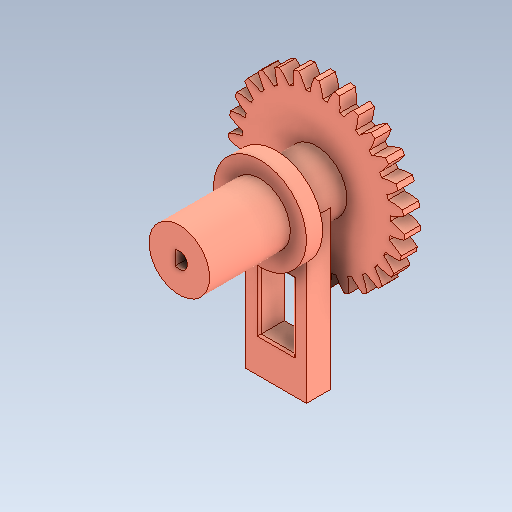
# Autodesk Inventor part: innerGear
Saved by Autodesk Inventor 2020.1 (Build 241239000, 239)
## iProperties
Created: 2020-01-18
Part Number: innerGear
Material: Generic
Document SubType Name: Modeling
Designer: Ali
Density: 1 g/cm^3
Appearance: Default
Author: Ali
Autodesk Inventor part; units mm, degrees
ref_plane "YZ Plane" through (0, 0, 0) normal (1, 0, 0) x (0, 1, 0)
sketch "Sketch1" plane through (0, 0, 0) normal (0, 0, 1) x (1, 0, 0)
  circle A0 centre (0, 0) radius 10
  dimension "d0" = 20
  constraints: 1 centre point, 1 coincident
  measures "d0" diameter of A0
extrude "Extrusion1" add sketch "Sketch1" along normal blind 2
sketch "Sketch2" plane through (0, 0, 2) normal (0, 0, 1) x (1, 0, 0)
  circle A0 centre (0, 0) radius 3.75
  dimension "d3" = 7.5
  constraints: 1 centre point, 1 coincident
  measures "d3" diameter of A0
extrude "Extrusion2" add sketch "Sketch2" along normal blind 17
ref_plane "Work Plane2" through (0, 0, 9) normal (0, 0, 1) x (1, 0, 0)
sketch "Sketch7" plane through (0, 0, 9) normal (0, 0, 1) x (1, 0, 0)
  circle A0 centre (0, 0) radius 3.75 projected
  circle A1 centre (0, 0) radius 5.75
  dimension "d27" = 2
  constraints: 1 centre point
  measures "d27" radial gap between concentric circles of A1 A0
extrude "Extrusion7" add sketch "Sketch7" against normal blind 2
sketch "Sketch8" plane through (0, 0, 7) normal (0, 0, -1) x (-1, 0, 0)
  circle A0 centre (0, 0) radius 5.75 projected
  circle A1 centre (0, 0) radius 3.75 projected
  circle A2 centre (0, 0) radius 5.75 construction
  line L0 (5.75, 0) -> (-5.75, 0) construction
  line L1 (-3.75, 0) -> (3.75, 0)
  line L2 (3.75, 0) -> (3.75, -19.5)
  line L3 (3.75, -19.5) -> (-3.75, -19.5)
  line L4 (-3.75, -19.5) -> (-3.75, 0)
  dimension "d31" = 19.5
  constraints: 10 end point, 2 horizontal, 2 parallel, 2 point on circle, 1 perpendicular, 1 point on line, 2 other
  measures "d31" distance of L1.end L2.end
extrude "Extrusion8" add sketch "Sketch8" along normal blind 3 contours L4 A1 L2 A0 | A0 L2 L3 L4 picked at (2.8343, -4.1874)
sketch "Sketch9" plane through (0, 0, 4) normal (0, 0, -1) x (-1, 0, 0)
  arc A0 (-3.75, -4.3589) -> (3.75, -4.3589) centre (0, 0) ccw projected
  line L0 (3.75, -19.5) -> (3.75, -4.3589) projected
  line L1 (-3.75, -19.5) -> (3.75, -19.5) projected
  line L2 (-3.75, -4.3589) -> (-3.75, -19.5) projected
  line L3 (-2, -7) -> (2, -7)
  line L4 (2, -7) -> (2, -15)
  line L5 (2, -15) -> (-2, -15)
  line L6 (-2, -15) -> (-2, -7)
  dimension "d34" = 2
  dimension "d35" = 4
  dimension "d36" = 8
  dimension "d37" = 7
  constraints: 8 end point, 2 parallel, 1 horizontal, 1 perpendicular
  measures "d34" distance from line of point (0, 0) L6
  measures "d35" distance of L4.end L5.end
  measures "d36" distance between parallel lines of L5 L3
  measures "d37" distance from line of point (0, 0) L3
extrude "Extrusion9" cut sketch "Sketch9" against normal up to surface (3 mm away) draft 2 contours L3 L4 L5 L6
fillet "Fillet2" radius 0.25 4 edges at (0, -15.1048, 7) (2.1048, -11, 7) (-2.1048, -11, 7) (0, -6.8952, 7)
sketch "Sketch10" plane through (0, 0, 19) normal (0, 0, 1) x (1, 0, 0)
  circle A0 centre (0, 0) radius 1
  circle A1 centre (0, 0) radius 3.75 projected
  line L0 (-0.5, 0.866) -> (-0.5, -0.866)
  point P0 (0, 1)
  point P1 (0, -1)
  dimension "d52" = 2
  dimension "d54" = 1.5
  constraints: 4 point on circle, 2 coincident, 2 end point, 1 centre point, 1 vertical
  measures "d52" diameter of A0
extrude "Extrusion10" cut sketch "Sketch10" against normal blind 5 contours A0 L0 picked at (0, 0)
ref_plane "Work Plane3" through (0, 0, 2) normal (0, 0, 1) x (1, 0, 0)
split "Split1" plane through (0, 0, 2) removes the side toward (0, 0, -1)
sketch "Sketch14" plane through (0, 0, 2) normal (0, 0, -1) x (-1, 0, 0)
  arc A0 (-2.8147, 10.5044) -> (-2.8899, 8.7212) centre (4.2594, 9.3128) ccw
  arc A1 (-2.8899, 8.7212) -> (-3.3921, 8.5384) centre (0, 0) ccw
  arc A2 (-3.3921, 8.5384) -> (-4.596, 9.8561) centre (-9.2491, 4.3961) ccw
  arc A3 (-4.596, 9.8561) -> (-5.1613, 9.5722) centre (0, 0) ccw
  arc A4 (-5.1613, 9.5722) -> (-4.8232, 7.8196) centre (1.9969, 10.0441) ccw
  arc A5 (-4.8232, 7.8196) -> (-5.2697, 7.526) centre (0, 0) ccw
  arc A6 (-5.2697, 7.526) -> (-6.7451, 8.5305) centre (-10.0136, 2.1447) ccw
  arc A7 (-6.7451, 8.5305) -> (-7.2297, 8.1239) centre (0, 0) ccw
  arc A8 (-7.2297, 8.1239) -> (-6.4965, 6.4965) centre (-0.3732, 10.2339) ccw
  arc A9 (-6.4965, 6.4965) -> (-6.8633, 6.1078) centre (0, 0) ccw
  arc A10 (-6.8633, 6.1078) -> (-8.5305, 6.7451) centre (-10.2382, -0.2224) ccw
  arc A11 (-8.5305, 6.7451) -> (-8.9083, 6.2376) centre (0, 0) ccw
  arc A12 (-8.9083, 6.2376) -> (-7.8196, 4.8232) centre (-2.7233, 9.8719) ccw
  arc A13 (-7.8196, 4.8232) -> (-8.0869, 4.3604) centre (0, 0) ccw
  arc A14 (-8.0869, 4.3604) -> (-9.8561, 4.596) centre (-9.911, -2.5775) ccw
  arc A15 (-9.8561, 4.596) -> (-10.1067, 4.0151) centre (0, 0) ccw
  arc A16 (-10.1067, 4.0151) -> (-8.7212, 2.8899) centre (-4.9265, 8.9778) ccw
  arc A17 (-8.7212, 2.8899) -> (-8.8744, 2.3779) centre (0, 0) ccw
  arc A18 (-8.8744, 2.3779) -> (-10.6503, 2.1991) centre (-9.0494, -4.7937) ccw
  arc A19 (-10.6503, 2.1991) -> (-10.7602, 1.5761) centre (0, 0) ccw
  arc A20 (-10.7602, 1.5761) -> (-9.1525, 0.8007) centre (-6.8641, 7.5997) ccw
  arc A21 (-9.1525, 0.8007) -> (-9.1836, 0.2672) centre (0, 0) ccw
  arc A22 (-9.1836, 0.2672) -> (-10.8704, -0.3163) centre (-7.7, -6.7514) ccw
  arc A23 (-10.8704, -0.3163) -> (-10.8336, -0.9478) centre (0, 0) ccw
  arc A24 (-10.8336, -0.9478) -> (-9.0905, -1.3316) centre (-8.4317, 5.8119) ccw
  arc A25 (-9.0905, -1.3316) -> (-8.9977, -1.8579) centre (0, 0) ccw
  arc A26 (-8.9977, -1.8579) -> (-10.5044, -2.8147) centre (-5.9354, -8.3452) ccw
  arc A27 (-10.5044, -2.8147) -> (-10.323, -3.4207) centre (0, 0) ccw
  arc A28 (-10.323, -3.4207) -> (-8.5384, -3.3921) centre (-9.5447, 3.7107) ccw
  arc A29 (-8.5384, -3.3921) -> (-8.3267, -3.8828) centre (0, 0) ccw
  arc A30 (-8.3267, -3.8828) -> (-9.5722, -5.1613) centre (-3.8509, -9.489) ccw
  arc A31 (-9.5722, -5.1613) -> (-9.2559, -5.7091) centre (0, 0) ccw
  arc A32 (-9.2559, -5.7091) -> (-7.526, -5.2697) centre (-10.1432, 1.4095) ccw
  arc A33 (-7.526, -5.2697) -> (-7.2068, -5.6984) centre (0, 0) ccw
  arc A34 (-7.2068, -5.6984) -> (-8.1239, -7.2297) centre (-1.5588, -10.1213) ccw
  arc A35 (-8.1239, -7.2297) -> (-7.6898, -7.6898) centre (0, 0) ccw
  arc A36 (-7.6898, -7.6898) -> (-6.1078, -6.8633) centre (-10.1948, -0.9676) ccw
  arc A37 (-6.1078, -6.8633) -> (-5.6984, -7.2068) centre (0, 0) ccw
  arc A38 (-5.6984, -7.2068) -> (-6.2376, -8.9083) centre (0.8174, -10.208) ccw
  arc A39 (-6.2376, -8.9083) -> (-5.7091, -9.2559) centre (0, 0) ccw
  arc A40 (-5.7091, -9.2559) -> (-4.3604, -8.0869) centre (-9.6969, -3.2927) ccw
  arc A41 (-4.3604, -8.0869) -> (-3.8828, -8.3267) centre (0, 0) ccw
  arc A42 (-3.8828, -8.3267) -> (-4.0151, -10.1067) centre (3.1495, -9.7443) ccw
  arc A43 (-4.0151, -10.1067) -> (-3.4207, -10.323) centre (0, 0) ccw
  arc A44 (-3.4207, -10.323) -> (-2.3779, -8.8744) centre (-8.6762, -5.4402) ccw
  arc A45 (-2.3779, -8.8744) -> (-1.8579, -8.9977) centre (0, 0) ccw
  arc A46 (-1.8579, -8.9977) -> (-1.5761, -10.7602) centre (5.3118, -8.7554) ccw
  arc A47 (-1.5761, -10.7602) -> (-0.9478, -10.8336) centre (0, 0) ccw
  arc A48 (-0.9478, -10.8336) -> (-0.2672, -9.1836) centre (-7.1877, -7.2944) ccw
  arc A49 (-0.2672, -9.1836) -> (0.2672, -9.1836) centre (0, 0) ccw
  arc A50 (0.2672, -9.1836) -> (0.9478, -10.8336) centre (7.1877, -7.2944) ccw
  arc A51 (0.9478, -10.8336) -> (1.5761, -10.7602) centre (0, 0) ccw
  arc A52 (1.5761, -10.7602) -> (1.8579, -8.9977) centre (-5.3118, -8.7554) ccw
  arc A53 (1.8579, -8.9977) -> (2.3779, -8.8744) centre (0, 0) ccw
  arc A54 (2.3779, -8.8744) -> (3.4207, -10.323) centre (8.6762, -5.4402) ccw
  arc A55 (3.4207, -10.323) -> (4.0151, -10.1067) centre (0, 0) ccw
  arc A56 (4.0151, -10.1067) -> (3.8828, -8.3267) centre (-3.1495, -9.7443) ccw
  arc A57 (3.8828, -8.3267) -> (4.3604, -8.0869) centre (0, 0) ccw
  arc A58 (4.3604, -8.0869) -> (5.7091, -9.2559) centre (9.6969, -3.2927) ccw
  arc A59 (5.7091, -9.2559) -> (6.2376, -8.9083) centre (0, 0) ccw
  arc A60 (6.2376, -8.9083) -> (5.6984, -7.2068) centre (-0.8174, -10.208) ccw
  arc A61 (5.6984, -7.2068) -> (6.1078, -6.8633) centre (0, 0) ccw
  arc A62 (6.1078, -6.8633) -> (7.6898, -7.6898) centre (10.1948, -0.9676) ccw
  arc A63 (7.6898, -7.6898) -> (8.1239, -7.2297) centre (0, 0) ccw
  arc A64 (8.1239, -7.2297) -> (7.2068, -5.6984) centre (1.5588, -10.1213) ccw
  arc A65 (7.2068, -5.6984) -> (7.526, -5.2697) centre (0, 0) ccw
  arc A66 (7.526, -5.2697) -> (9.2559, -5.7091) centre (10.1432, 1.4095) ccw
  arc A67 (9.2559, -5.7091) -> (9.5722, -5.1613) centre (0, 0) ccw
  arc A68 (9.5722, -5.1613) -> (8.3267, -3.8828) centre (3.8509, -9.489) ccw
  arc A69 (8.3267, -3.8828) -> (8.5384, -3.3921) centre (0, 0) ccw
  arc A70 (8.5384, -3.3921) -> (10.323, -3.4207) centre (9.5447, 3.7107) ccw
  arc A71 (10.323, -3.4207) -> (10.5044, -2.8147) centre (0, 0) ccw
  arc A72 (10.5044, -2.8147) -> (8.9977, -1.8579) centre (5.9354, -8.3452) ccw
  arc A73 (8.9977, -1.8579) -> (9.0905, -1.3316) centre (0, 0) ccw
  arc A74 (9.0905, -1.3316) -> (10.8336, -0.9478) centre (8.4317, 5.8119) ccw
  arc A75 (10.8336, -0.9478) -> (10.8704, -0.3163) centre (0, 0) ccw
  arc A76 (10.8704, -0.3163) -> (9.1836, 0.2672) centre (7.7, -6.7514) ccw
  arc A77 (9.1836, 0.2672) -> (9.1525, 0.8007) centre (0, 0) ccw
  arc A78 (9.1525, 0.8007) -> (10.7602, 1.5761) centre (6.8641, 7.5997) ccw
  arc A79 (10.7602, 1.5761) -> (10.6503, 2.1991) centre (0, 0) ccw
  arc A80 (10.6503, 2.1991) -> (8.8744, 2.3779) centre (9.0494, -4.7937) ccw
  arc A81 (8.8744, 2.3779) -> (8.7212, 2.8899) centre (0, 0) ccw
  arc A82 (8.7212, 2.8899) -> (10.1067, 4.0151) centre (4.9265, 8.9778) ccw
  arc A83 (10.1067, 4.0151) -> (9.8561, 4.596) centre (0, 0) ccw
  arc A84 (9.8561, 4.596) -> (8.0869, 4.3604) centre (9.911, -2.5775) ccw
  arc A85 (8.0869, 4.3604) -> (7.8196, 4.8232) centre (0, 0) ccw
  arc A86 (7.8196, 4.8232) -> (8.9083, 6.2376) centre (2.7233, 9.8719) ccw
  arc A87 (8.9083, 6.2376) -> (8.5305, 6.7451) centre (0, 0) ccw
  arc A88 (8.5305, 6.7451) -> (6.8633, 6.1078) centre (10.2382, -0.2224) ccw
  arc A89 (6.8633, 6.1078) -> (6.4965, 6.4965) centre (0, 0) ccw
  arc A90 (6.4965, 6.4965) -> (7.2297, 8.1239) centre (0.3732, 10.2339) ccw
  arc A91 (7.2297, 8.1239) -> (6.7451, 8.5305) centre (0, 0) ccw
  arc A92 (6.7451, 8.5305) -> (5.2697, 7.526) centre (10.0136, 2.1447) ccw
  arc A93 (5.2697, 7.526) -> (4.8232, 7.8196) centre (0, 0) ccw
  arc A94 (4.8232, 7.8196) -> (5.1613, 9.5722) centre (-1.9969, 10.0441) ccw
  arc A95 (5.1613, 9.5722) -> (4.596, 9.8561) centre (0, 0) ccw
  arc A96 (4.596, 9.8561) -> (3.3921, 8.5384) centre (9.2491, 4.3961) ccw
  arc A97 (3.3921, 8.5384) -> (2.8899, 8.7212) centre (0, 0) ccw
  arc A98 (2.8899, 8.7212) -> (2.8147, 10.5044) centre (-4.2594, 9.3128) ccw
  arc A99 (2.8147, 10.5044) -> (2.1991, 10.6503) centre (0, 0) ccw
  arc A100 (2.1991, 10.6503) -> (1.3316, 9.0905) centre (7.9859, 6.4106) ccw
  arc A101 (1.3316, 9.0905) -> (0.8007, 9.1525) centre (0, 0) ccw
  arc A102 (0.8007, 9.1525) -> (0.3163, 10.8704) centre (-6.2923, 8.0795) ccw
  arc A103 (0.3163, 10.8704) -> (-0.3163, 10.8704) centre (0, 0) ccw
  arc A104 (-0.3163, 10.8704) -> (-0.8007, 9.1525) centre (6.2923, 8.0795) ccw
  arc A105 (-0.8007, 9.1525) -> (-1.3316, 9.0905) centre (0, 0) ccw
  arc A106 (-1.3316, 9.0905) -> (-2.1991, 10.6503) centre (-7.9859, 6.4106) ccw
  arc A107 (-2.1991, 10.6503) -> (-2.8147, 10.5044) centre (0, 0) ccw
  constraints: 216 point on circle, 108 centre point
extrude "Extrusion14" add sketch "Sketch14" along normal blind 2
equation "\"d1\" = IG_gearThickness"
equation "\"d3\" = IG_shaftDiameter"
equation "\"d4\" = IG_shaftLength"
equation "\"Wheel_Related_W_\" = 0"
equation "\"W_innerDepth\" = 4"
equation "\"W_wallThickness\" = 2"
equation "\"W_holesClearance\" = 0.3"
equation "\"W_outerGearHoleDiameter\" = 5.3"
equation "\"W_innerGearHoleDiameter\" = 10.1"
equation "\"TempSpotReserved7\" = 0"
equation "\"TempSpotReserved8\" = 0"
equation "\"TempSpotReserved9\" = 0"
equation "\"TempSpotReserved10\" = 0"
equation "\"TempSpotReserved11\" = 0"
equation "\"TempSpotReserved12\" = 0"
equation "\"TempSpotReserved13\" = 0"
equation "\"TempSpotReserved14\" = 0"
equation "\"TempSpotReserved15\" = 0"
equation "\"TempSpotReserved16\" = 0"
equation "\"TempSpotReserved17\" = 0"
equation "\"TempSpotReserved18\" = 0"
equation "\"TempSpotReserved19\" = 0"
equation "\"TempSpotReserved20\" = 0"
equation "\"Inner_Gear_Related_IG_\" = 0"
equation "\"IG_shaftDiameter\" = 7.5"
equation "\"IG_shaftLength\" = 17"
equation "\"IG_gearThickness\" = 2"
equation "\"TempSpotReserved25\" = 0"
equation "\"TempSpotReserved26\" = 0"
equation "\"TempSpotReserved27\" = 0"
equation "\"TempSpotReserved28\" = 0"
equation "\"TempSpotReserved29\" = 0"
equation "\"TempSpotReserved30\" = 0"
equation "\"TempSpotReserved31\" = 0"
equation "\"TempSpotReserved32\" = 0"
equation "\"TempSpotReserved33\" = 0"
equation "\"TempSpotReserved34\" = 0"
equation "\"TempSpotReserved35\" = 0"
equation "\"TempSpotReserved36\" = 0"
equation "\"TempSpotReserved37\" = 0"
equation "\"TempSpotReserved38\" = 0"
equation "\"TempSpotReserved39\" = 0"
equation "\"TempSpotReserved40\" = 0"
equation "\"Outer_Gear_Related_OG_\" = 0"
equation "\"OG_distanceFromCenter\" = 22.5"
equation "\"OG_shaftDiameter\" = 5"
equation "\"OG_gearDiameter\" = 25"
equation "\"OG_shaftLength\" = 9"
equation "\"OG_gearThickness\" = 2"
equation "\"TempSpotReserved47\" = 0"
equation "\"TempSpotReserved48\" = 0"
equation "\"TempSpotReserved49\" = 0"
equation "\"TempSpotReserved50\" = 0"
equation "\"TempSpotReserved51\" = 0"
equation "\"TempSpotReserved52\" = 0"
equation "\"TempSpotReserved53\" = 0"
equation "\"TempSpotReserved54\" = 0"
equation "\"TempSpotReserved55\" = 0"
equation "\"TempSpotReserved56\" = 0"
equation "\"TempSpotReserved57\" = 0"
equation "\"TempSpotReserved58\" = 0"
equation "\"TempSpotReserved59\" = 0"
equation "\"TempSpotReserved60\" = 0"
equation "\"Leg_Extensions_Related_LE_\" = 0"
equation "\"LE_baseDiameter\" = 5"
equation "\"LE_maxLength\" = 23.67256"
equation "\"LE_thickness\" = 2.5"
equation "\"IG_ratioToOuterGear\" = 1.25"
equation "\"B_bearingThickness\" = 1"
equation "\"TempSpotReserved43\" = 0"
equation "\"TempSpotReserved45\" = 0"
equation "\"Thisisatest\" = 25.4"
equation "\"TempSpotReserved46\" = 0"
equation "\"TempSpotReserved44\" = 0"
equation "\"LE_offsetAboveOuterGear\" = 0"
equation "\"Bearing_Related_B_\" = 0"
equation "\"TempSpotReserved42\" = 0"
equation "\"OG_skirtOffset\" = 5"
equation "\"OG_skirtThickness\" = 1"
equation "\"IG_skirtThickness\" = 2"
equation "\"IG_extentionLength\" = 19.5"
equation "\"IG_extentionThickness\" = 3"
equation "\"IG_slitWidth\" = 4"
equation "\"IG_slitlength\" = 8"
equation "\"IG_slitDistanceFromCenterHole\" = 7"
equation "\"IG_slitClearance\" = 0.2"
equation "\"Reserved_10\" = 0"
equation "\"Reserved_9\" = 0"
equation "\"Reserved_11\" = 0"
equation "\"Reserved_12\" = 0"
equation "\"Reserved_8\" = 0"
equation "\"Reserved_7\" = 0"
equation "\"Reserved_26\" = 0"
equation "\"Reserved_20\" = 0"
equation "\"Reserved_22\" = 0"
equation "\"Reserved_23\" = 0"
equation "\"Reserved_25\" = 0"
equation "\"Reserved_24\" = 0"
equation "\"Reserved_21\" = 0"
equation "\"Reserved_19\" = 0"
equation "\"Reserved_27\" = 0"
equation "\"Reserved_14\" = 0"
equation "\"Reserved_15\" = 0"
equation "\"Reserved_16\" = 0"
equation "\"Reserved_13\" = 0"
equation "\"Reserved_17\" = 0"
equation "\"Reserved_18\" = 0"
equation "\"Bearing_Related_BR_\" = 0"
equation "\"BR_bearingThickness\" = 1"
equation "\"Block_Related_BL_\" = 0"
equation "\"BL_width\" = 3.8"
equation "\"BL_length\" = 7.8"
equation "\"W_filletRadius\" = 0.25"
equation "\"W_extrutsionTaperAngle\" = 2deg"
equation "\"OG_protrudeDistance\" = 3"
equation "\"IG_dAxleCircleDiameter\" = 2"
equation "\"IG_dAxleShort\" = 1.5"
equation "\"IG_dAxleDepth\" = 5"
equation "\"IG_gearRatio\" = 1.25"
body "Solid1"
